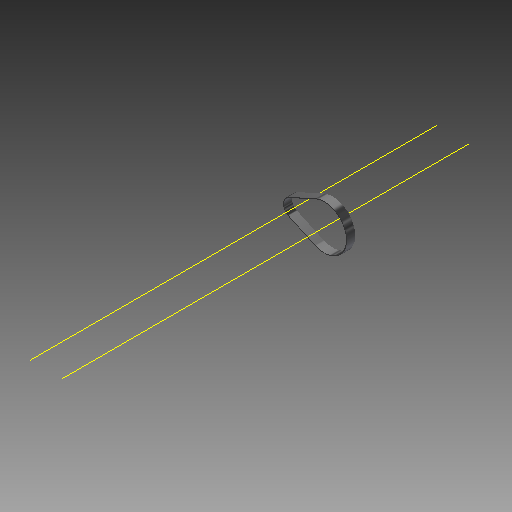
# Autodesk Inventor part: Zahnriemen
Saved by Autodesk Inventor 2018.3 (Build 223284000, 284)
## iProperties
Created: 2018-07-27
Part Number: Zahnriemen
Material: Rubber
Document SubType Name: Modeling
Designer: JochenAlt
Density: 1 g/cm^3
Appearance: Rubber - Black - Version 1.1
Author: JochenAlt
Autodesk Inventor part; units mm, degrees
ref_plane "YZ Plane" through (0, 0, 0) normal (1, 0, 0) x (0, 1, 0)
ref_plane "XZ Plane" through (0, 0, 0) normal (0, 1, 0) x (-1, 0, 0)
ref_plane "XY Plane" through (0, 0, 0) normal (0, 0, 1) x (1, 0, 0)
sketch "Skizzenpfad" plane through (0, 0, 0) normal (0, 0, 1) x (1, 0, 0)
  arc A0 (-102.6447, 5.7908) -> (-102.6447, -5.7908) centre (-100, 0) ccw
  arc A1 (-83.6255, -14.4771) -> (-83.6255, 14.4771) centre (-77.0137, 0) ccw
  line L0 (-83.6255, -14.4771) -> (-102.6447, -5.7908)
  line L1 (-102.6447, 5.7908) -> (-83.6255, 14.4771)
  constraints: 4 end point, 4 point on circle, 2 centre point
ref_plane "Querschnittsebene" through (-102.6447, -5.7908, 0) normal (0.9096233, -0.415434, 0) x (0, 0, 1)
ref_plane "Arbeitsebene2" through (-100, 0, 0) normal (-1, 0, 0) x (0, 0, 1)
ref_plane "Arbeitsebene3" through (-77.0137, 0, 0) normal (-0.9510566, -0.3090168, 0) x (0, 0, 1)
sketch "Querschnitt" plane through (-102.6447, -5.7908, 0) normal (0.9096233, -0.415434, 0) x (0, 0, 1)
  line L0 (-3, 0.3) -> (3, 0.3)
  line L1 (3, 0.3) -> (3, -0.3)
  line L2 (3, -0.3) -> (-3, -0.3)
  line L3 (-3, -0.3) -> (-3, 0.3)
  line L4 (-3, 0) -> (3, 0) construction
  point P0 (0, 0)
  point P1 (0, 0)
  dimension "d0" = 6
  dimension "d4" = 0.3
  dimension "d5" = 0.3
  constraints: 10 end point, 3 midpoint, 2 parallel, 1 coincident, 1 horizontal, 1 perpendicular, 1 other
  measures "d0" distance between parallel lines of L1 L3
  measures "d4" distance between parallel lines of L2 L4
  measures "d5" distance between parallel lines of L4 L0
sweep "Riemen" add profiles "Querschnitt" path "Skizzenpfad" path curves L1 A1 L0 A0
equation "\"d0\" = da_B"
equation "\"d4\" = da_a"
equation "\"d5\" = da_a2"
equation "\"da_B\" = 6"
equation "\"da_pb\" = 2.5"
equation "\"da_a\" = 0.3"
equation "\"da_S\" = 1.5"
equation "\"da_Beta\" = 20deg"
equation "\"da_Ht\" = 0.7"
equation "\"da_H\" = 1.3"
equation "\"da_a2\" = 0.3"
body "Solid1"
